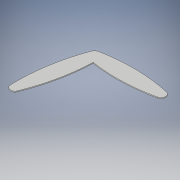
# Autodesk Inventor part: side
Saved by Autodesk Inventor 2019 (Build 230136000, 136)
## iProperties
Created: 2018-12-28
Part Number: side
Material: Generic
Document SubType Name: Modeling
Designer: gaincarlo
Density: 1 g/cm^3
Appearance: Default
Author: gaincarlo
Autodesk Inventor part; units mm, degrees
ref_plane "YZ Plane" through (0, 0, 0) normal (1, 0, 0) x (0, 1, 0)
ref_plane "XZ Plane" through (0, 0, 0) normal (0, 1, 0) x (-1, 0, 0)
ref_plane "XY Plane" through (0, 0, 0) normal (0, 0, 1) x (1, 0, 0)
sketch "Sketch1" plane through (0, 0, 0) normal (0, 1, 0) x (-1, 0, 0)
  line L0 (0, 0) -> (-700, 0) construction
  line L1 (-700, 0) -> (-700, 600) construction
  line L2 (-700, 600) -> (0, 600) construction
  line L3 (0, 600) -> (0, 0) construction
  circle A0 centre (0, 600) radius 40
  line L4 (0, 600) -> (-105.7962, 0) construction
  circle A1 centre (-105.7962, 0) radius 50
  line L5 (1496.5572, 0) -> (-37.1273, 614.8851) construction
  circle A2 centre (-700, 0) radius 40
  circle A3 centre (-1611.5159, 548.0371) radius 1652.3534 construction
  line L6 (-1611.5159, 548.0371) -> (-58.8116, -17.101) construction
  line L7 (-1611.5159, 548.0371) -> (39.9792, 601.2891) construction
  line L8 (1496.5572, 0) -> (-1611.5159, 548.0371) construction
  line L9 (1496.5572, 0) -> (-155.7962, 0) construction
  arc A4 (-58.8116, -17.101) -> (39.9792, 601.2891) centre (-1611.5159, 548.0371) ccw
  arc A5 (-37.1273, 614.8851) -> (-155.7962, 0) centre (1496.5572, 0) ccw
  line L10 (-378.4115, -1424.1422) -> (-96.3957, 49.1084) construction
  line L11 (-708.8106, 39.0176) -> (-378.4115, -1424.1422) construction
  arc A6 (-708.8106, -39.0176) -> (-96.3957, -49.1084) centre (-378.4115, 1424.1422) ccw
  arc A7 (92.5652, 0) -> (-849.3883, 0) centre (-378.4115, 1424.1422) ccw construction
  arc A8 (-849.3883, 0) -> (0, 27.3415) centre (-378.4115, -1424.1422) ccw construction
  arc A9 (-40.1065, 37.2099) -> (-708.8106, 39.0176) centre (-378.4115, -1424.1422) ccw
  point P0 (-106.0172, 49.9995)
  point P1 (-701.1693, 39.9829)
  point P2 (-106.0172, -49.9995)
  point P3 (-701.1693, -39.9829)
  dimension "d0" = 700
  dimension "d1" = 600
  dimension "d3" = 80
  dimension "d5" = 10
  dimension "d7" = 100
  dimension "d9" = 80
  constraints: 29 point on circle, 24 end point, 10 centre point, 8 point on line, 3 coincident, 2 parallel, 2 perpendicular, 1 collinear, 1 horizontal, 1 symmetric about line
  measures "d0" distance of L1.end L2.end
  measures "d1" distance of L0.end L1.end
  measures "d3" diameter of A0
  measures "d5" angle of L3 L4
  measures "d7" diameter of A1
  measures "d9" diameter of A2
extrude "Extrusion2" add sketch "Sketch1" along normal blind 8
body "Solid2"
